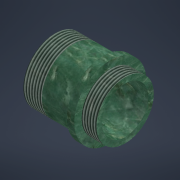
# Autodesk Inventor part: 027
Saved by Autodesk Inventor 2022 (Build 260153000, 153)
## iProperties
Created: 2022-04-04
Part Number: 027
Material: Aluminum 6061
Document SubType Name: Modeling
Designer: Vinicius Miguel
Density: 2.7 g/cm^3
Appearance: Smooth - Dark Forest Green
Mass: 41.2435 g
Surface Area: 84.7602 cm^2
Volume: 15.2754 cm^3
Author: Vinicius Miguel
Autodesk Inventor part; units mm, degrees
ref_plane "YZ Plane" through (0, 0, 0) normal (1, 0, 0) x (0, 1, 0)
ref_plane "XZ Plane" through (0, 0, 0) normal (0, 1, 0) x (-1, 0, 0)
ref_plane "XY Plane" through (0, 0, 0) normal (0, 0, 1) x (1, 0, 0)
sketch "Sketch1" plane through (0, 0, 0) normal (0, 1, 0) x (-1, 0, 0)
  line L0 (0, 0) -> (-9.3015, 0)
  line L1 (25, -12.5) -> (-8, -12.5)
  line L2 (-8, -12.5) -> (-8, -15.5)
  line L3 (-8, -15.5) -> (0, -15.5)
  line L4 (0, -15.5) -> (0, -19.5)
  line L5 (0, -19.5) -> (4, -19.5)
  line L6 (0, -16.25) -> (1.2, -16.25)
  line L7 (1.2, -16.25) -> (1.2, -18.25)
  line L8 (1.2, -18.25) -> (0, -18.25)
  line L9 (4, -19.5) -> (4, -17)
  line L10 (4, -17) -> (30, -17)
  line L11 (30, -17) -> (30, -13.7)
  line L12 (30, -13.7) -> (25, -13.7)
  line L13 (25, -13.7) -> (25, -12.5)
  dimension "d0" = 25
  dimension "d1" = 8
  dimension "d2" = 25
  dimension "d3" = 3
  dimension "d4" = 4
  dimension "d5" = 2
  dimension "d6" = 1.2
  dimension "d7" = 1.25
  dimension "d8" = 4.5
  dimension "d9" = 5
  dimension "d10" = 1.2
  dimension "d11" = 4
  constraints: 28 end point, 10 perpendicular, 3 horizontal, 2 point on line, 1 vertical, 1 vertical alignment
  measures "d0" horizontal distance of L1.start L0.start
  measures "d1" distance of L2.end L3.end
  measures "d2" diameter of L1 L0
  measures "d3" distance of L1.end L2.end
  measures "d4" distance of L3.end L4.end
  measures "d5" distance of L6.end L7.end
  measures "d6" distance of L6.start L6.end
  measures "d7" distance between parallel lines of L5 L8
  measures "d8" distance between parallel lines of L10 L1
  measures "d9" distance of L11.end L12.end
  measures "d10" distance of L12.end L1.start
  measures "d11" distance of L4.end L5.end
revolve "Revolution1" add sketch "Sketch1" angle 360 about axis through (0, 0, 0) along (1, 0, 0)
thread "Thread1" size "M32x1.5" class "6g" standard "ANSI Metric M Profile" length 10
thread "Thread2" size "M28x1" class "6H" standard "ANSI Metric M Profile" length 10
thread "Thread3" size "M35x1.5" class "6g" standard "ANSI Metric M Profile" length 10
body "Solid1"
